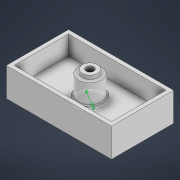
# Autodesk Inventor part: Servoverbindung_Konzept
Saved by Autodesk Inventor 2021 (Build 250183000, 183)
## iProperties
Created: 2021-01-13
Part Number: Servoverbindung_Konzept
Material: Generisch
Document SubType Name: Modeling
Designer: Ctroi
Density: 1 g/cm^3
Appearance: Vorgabe
Author: Ctroi
Autodesk Inventor part; units mm, degrees
ref_plane "YZ Plane" through (0, 0, 0) normal (1, 0, 0) x (0, 1, 0)
ref_plane "XZ Plane" through (0, 0, 0) normal (0, 1, 0) x (-1, 0, 0)
ref_plane "XY Plane" through (0, 0, 0) normal (0, 0, 1) x (1, 0, 0)
sketch "Skizze1" plane through (0, 0, 0) normal (0, 1, 0) x (-1, 0, 0)
  line L0 (-27.5, -16.25) -> (27.5, -16.25)
  line L1 (27.5, -16.25) -> (27.5, 16.25)
  line L2 (27.5, 16.25) -> (-27.5, 16.25)
  line L3 (-27.5, 16.25) -> (-27.5, -16.25)
  line L4 (-38.5, 0) -> (38.5, 0) projected
  line L5 (0, -22.75) -> (0, 22.75) projected
  point P0 (0, 0)
  dimension "d0" = 55
  dimension "d1" = 32.5
  constraints: 8 end point, 2 parallel, 1 horizontal, 1 perpendicular, 2 other
  measures "d0" distance of L1.end L2.end
  measures "d1" distance of L0.end L1.end
extrude "Extrusion1" add sketch "Skizze1" along normal blind 5
sketch "Skizze5" plane through (0, 5, 0) normal (0, 1, 0) x (1, 0, 0)
  line L0 (27.5, 16.25) -> (-27.5, 16.25) projected
  line L1 (27.5, -16.25) -> (27.5, 16.25) projected
  line L2 (-27.5, 16.25) -> (27.5, 16.25)
  line L3 (27.5, 16.25) -> (27.5, -16.25)
  line L4 (27.5, -16.25) -> (-27.5, -16.25)
  line L5 (-27.5, -16.25) -> (-27.5, 16.25)
  line L6 (-25.5, 14.25) -> (25.5, 14.25)
  line L7 (25.5, 14.25) -> (25.5, -14.25)
  line L8 (25.5, -14.25) -> (-25.5, -14.25)
  line L9 (-25.5, -14.25) -> (-25.5, 14.25)
  point P0 (0, 0)
  dimension "d14" = 2
  constraints: 16 end point, 4 parallel, 2 perpendicular, 1 horizontal, 3 other
  measures "d14" distance between parallel lines of L5 L9
extrude "Extrusion5" add sketch "Skizze5" along normal blind 10
sketch "Skizze6" plane through (0, 5, 0) normal (0, 1, 0) x (1, 0, 0)
  circle A0 centre (0, 0) radius 6
  circle A1 centre (0, 0) radius 7
  dimension "d17" = 12
  dimension "d18" = 14
  constraints: 2 centre point, 2 coincident
  measures "d17" diameter of A0
  measures "d18" diameter of A1
extrude "Extrusion6" add sketch "Skizze6" along normal blind 2
extrude "Extrusion7" add sketch "Skizze6" along normal blind 12 contours A0
sketch "Skizze8" plane through (0, 17, 0) normal (0, 1, 0) x (1, 0, 0)
  circle A0 centre (0, 0) radius 3.95
  dimension "d23" = 7.9
  constraints: 1 centre point, 1 coincident
  measures "d23" diameter of A0
extrude "Extrusion8" add sketch "Skizze8" along normal blind 2
sketch "Skizze9" plane through (0, 19, 0) normal (0, 1, 0) x (1, 0, 0)
  circle A0 centre (0, 0) radius 2
  dimension "d26" = 4
  constraints: 1 centre point, 1 coincident
  measures "d26" diameter of A0
extrude "Extrusion9" cut sketch "Skizze9" against normal blind 4
